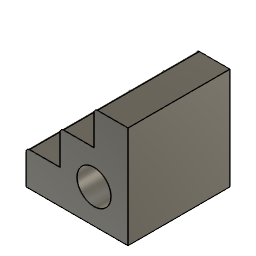
auv_q_one (Autodesk Fusion 360 design; units mm, degrees)
part number: 2026-04-12-23-27-13-794
Autodesk Fusion 360 part; units mm, degrees
sketch "Sketch1" plane through (0, 0, 0) normal (0, 1, 0) x (1, 0, 0)
  line L0 (0, 0) -> (-45, 0)
  line L1 (-50, 5) -> (-50, 50)
  line L2 (-50, 50) -> (-95, 50)
  line L3 (-100, 55) -> (-100, 100)
  line L4 (-100, 100) -> (-145, 100)
  line L5 (-150, 105) -> (-150, 150)
  line L6 (-150, 150) -> (0, 150)
  line L7 (0, 150) -> (0, 0)
  line L8 (-50, 50) -> (-50, 100)
  circle A0 centre (-50, 100) radius 25
  arc A1 (-50, 5) -> (-45, 0) centre (-45, 5) ccw
  arc A2 (-100, 55) -> (-95, 50) centre (-95, 55) ccw
  arc A3 (-150, 105) -> (-145, 100) centre (-145, 105) ccw
  point P0 (-50, 0)
  point P1 (-100, 50)
  point P2 (-150, 100)
  dimension "d1" = 50
  dimension "d2" = 50
  dimension "d3" = 50
  dimension "d4" = 50
  dimension "d5" = 50
  dimension "d6" = 50
  dimension "d7" = 50
  dimension "d8" = 5
  dimension "d9" = 5
  dimension "d10" = 5
  constraint coincident L0.start L7.end
  constraint horizontal L0
  constraint perpendicular L0 L1
  constraint perpendicular L1 L2
  constraint perpendicular L2 L3
  constraint perpendicular L3 L4
  constraint perpendicular L4 L5
  constraint perpendicular L5 L6
  constraint perpendicular L0 L7
  constraint perpendicular L2 L8
  constraint coincident P0 L0
  constraint coincident P0 L1
  constraint tangent L0 A1
  constraint tangent L1 A1
  constraint coincident P1 L2
  constraint coincident P1 L3
  constraint tangent L2 A2
  constraint tangent L3 A2
  constraint coincident P2 L4
  constraint coincident P2 L5
  constraint tangent L4 A3
  constraint tangent L5 A3
  measures "d1" distance of L0.start P0
  measures "d2" distance of P0 L1.end
  measures "d3" distance of L1.end P1
  measures "d4" distance of P1 L3.end
  measures "d5" distance of L3.end P2
  measures "d6" distance of P2 L5.end
  measures "d7" diameter of A0
  measures "d8" radius of A1
  measures "d9" radius of A2
  measures "d10" radius of A3
extrude "Extrude1" add sketch "Sketch1" along normal blind 150
